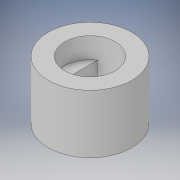
# Autodesk Inventor part: test_axis
Saved by Autodesk Inventor 2019 (Build 230136000, 136)
## iProperties
Created: 2019-09-12
Part Number: test_axis
Material: Generic
Document SubType Name: Modeling
Designer: assman
Density: 1 g/cm^3
Appearance: Default
Author: assman
## iProperties of the stored document test_axis_3DPrint.ipt
Created: 2019-09-12
Part Number: test_axis_3DPrint
Material: Generic
Document SubType Name: Modeling
Designer: assman
Density: 1 g/cm^3
Appearance: Default
Author: assman
Autodesk Inventor part; units mm, degrees
ref_plane "YZ Plane" through (0, 0, 0) normal (1, 0, 0) x (0, 1, 0)
ref_plane "XZ Plane" through (0, 0, 0) normal (0, 1, 0) x (-1, 0, 0)
ref_plane "XY Plane" through (0, 0, 0) normal (0, 0, 1) x (1, 0, 0)
sketch "Sketch1" plane through (0, 0, 0) normal (0, 1, 0) x (-1, 0, 0)
  circle A0 centre (0, 0) radius 5
  dimension "d0" = 10
  constraints: 1 centre point, 1 coincident
  measures "d0" diameter of A0
extrude "Extrusion1" add sketch "Sketch1" along normal blind 15
sketch "Sketch2" plane through (0, 15, 0) normal (0, 1, 0) x (1, 0, 0)
  circle A0 centre (0, 0) radius 3.025
  dimension "d3" = 6.05
  constraints: 1 centre point, 1 coincident
  measures "d3" diameter of A0
extrude "Extrusion2" cut sketch "Sketch2" against normal blind 12.5
sketch "Sketch3" plane through (0, 2.5, 0) normal (0, 1, 0) x (1, 0, 0)
  circle A0 centre (0, 0) radius 3.025 construction
  line L0 (-1.65, -3.3431) -> (-1.65, 4.0859) construction
  arc A1 (-1.65, 2.5354) -> (-1.65, -2.5354) centre (0, 0) ccw
  line L1 (-1.65, -2.5354) -> (-1.65, 2.5354)
  dimension "d6" = 1.65
  constraints: 4 end point, 4 point on circle, 2 point on line, 1 centre point, 1 coincident, 1 collinear, 1 vertical
  measures "d6" distance from line of point (0, 0) L0
extrude "Extrusion3" add sketch "Sketch3" along normal blind 10
sketch "Sketch4" plane through (0, 0, 0) normal (0, -1, 0) x (1, 0, 0)
  circle A0 centre (0, 0) radius 5 projected
extrude "Extrusion4" cut sketch "Sketch4" against normal blind 8
body "Solid1"
